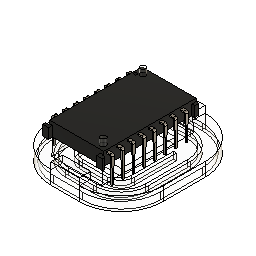
PMW3360 v12 (Autodesk Fusion 360 design; units mm, degrees)
Autodesk Fusion 360 part; units mm, degrees
sketch "Sketch1" plane through (0, 0, 0) normal (0, 0, 1) x (1, 0, 0) in component "Chip"
  line L0 (-4.55, 7.18) -> (4.55, 7.18)
  line L1 (4.55, 7.18) -> (4.55, -8.32)
  line L2 (4.55, -8.32) -> (-4.55, -8.32)
  line L3 (-4.55, -8.32) -> (-4.55, 7.18)
  line L4 (0, 7.18) -> (0, -8.32) construction
  dimension "d1" = 9.1
  dimension "d3" = 7.18
  dimension "d4" = 15.5
  constraint horizontal L0
  constraint vertical L1
  constraint horizontal L2
  constraint vertical L3
  constraint midpoint L0 L4.start
  constraint coincident L2 L4.end
  constraint vertical L4
  constraint coincident origin L4
  constraint coincident L4 origin
  measures "d1" distance of L0.start L0.end
  measures "d3" distance of L0 origin
  measures "d4" distance of L0.end L1.end
extrude "Extrude1" add sketch "Sketch1" against normal blind 0.5 makes body 1 in component "Chip"
sketch "Sketch2" plane through (0, 0, -0.5) normal (0, 0, -1) x (1, 0, 0) in component "Chip"
  line L0 (-4.55, 8.32) -> (4.55, 8.32)
  line L1 (4.55, 8.32) -> (4.55, -7.18)
  line L2 (4.55, -7.18) -> (-4.55, -7.18)
  line L3 (-4.55, -7.18) -> (-4.55, 8.32)
  line L4 (4.55, -7.18) -> (5.05, -7.18)
  line L5 (5.05, -7.18) -> (5.05, -6.48)
  line L6 (5.05, -6.48) -> (4.55, -6.48)
  line L7 (-4.55, -7.18) -> (-5.05, -7.18)
  line L8 (-5.05, -7.18) -> (-5.05, -6.68)
  line L9 (-4.85, -6.48) -> (-4.55, -6.48)
  line L10 (-4.55, -7.18) -> (-4.55, -6.48) construction
  line L11 (-5.05, -6.68) -> (-4.85, -6.48)
  line L12 (-4.55, 8.32) -> (-4.55, 8.52)
  line L13 (-4.55, 8.52) -> (-5.05, 8.52)
  line L14 (-5.05, 8.52) -> (-5.05, 9.02)
  line L15 (-5.05, 9.02) -> (-4.05, 9.02)
  line L16 (-4.05, 9.02) -> (-4.05, 8.32)
  line L17 (4.05, 8.32) -> (4.05, 9.02)
  line L18 (4.05, 9.02) -> (5.05, 9.02)
  line L19 (5.05, 9.02) -> (5.05, 8.72)
  line L20 (5.05, 8.72) -> (4.85, 8.52)
  line L21 (4.85, 8.52) -> (4.55, 8.52)
  line L22 (4.55, 8.52) -> (4.55, 8.32)
  dimension "d7" = 0.5
  dimension "d8" = 0.7
  dimension "d11" = 0.5
  dimension "d12" = 0.7
  dimension "d13" = 135
  dimension "d14" = 0.3
  dimension "d15" = 0.5
  dimension "d16" = 0.5
  dimension "d17" = 1
  dimension "d18" = 0.7
  dimension "d19" = 0.7
  dimension "d20" = 0.5
  dimension "d21" = 1
  dimension "d22" = 0.5
  dimension "d23" = 135
  dimension "d24" = 0.3
  constraint coincident L1.end L2.start
  constraint perpendicular L1 L4
  constraint perpendicular L4 L5
  constraint coincident L1 L6.end
  constraint perpendicular L1 L6
  constraint perpendicular L3 L7
  constraint perpendicular L7 L8
  constraint coincident L2.end L3.start
  constraint coincident L3 L9.end
  constraint perpendicular L3 L9
  constraint coincident L0.start L3.end
  constraint perpendicular L0 L12
  constraint perpendicular L3 L13
  constraint perpendicular L13 L14
  constraint perpendicular L14 L15
  constraint coincident L0 L16.end
  constraint perpendicular L0 L16
  constraint coincident L0 L17.start
  constraint perpendicular L0 L17
  constraint perpendicular L17 L18
  constraint perpendicular L18 L19
  constraint perpendicular L19 L21
  constraint coincident L0.end L1.start
  constraint vertical L22
  measures "d7" distance of L1.end L4.end
  measures "d8" distance of L4.end L5.end
  measures "d11" distance of L2.end L7.end
  measures "d12" distance of L2.end L9.end
  measures "d13" angle of L9 L11
  measures "d14" distance of L9.end L9.start
  measures "d15" distance of L12 L16
  measures "d16" distance of L13.end L14.end
  measures "d17" distance of L14.end L15.end
  measures "d18" distance of L15.end L16.end
  measures "d19" distance of L17.start L17.end
  measures "d20" distance of L18 L21
  measures "d21" distance of L17.end L18.end
  measures "d22" distance of L17 L22
  measures "d23" angle of L20 L21
  measures "d24" distance of L18.end L19.end
extrude "Extrude2" add sketch "Sketch2" along normal blind 1.71 bodies 1 in component "Chip"
ref_plane "WorkPlane1" through (0, 5.66, -1.105) normal (0, 1, 0) x (1, 0, 0) in component "Chip"
sketch "Sketch1 (2)" plane through (0, 5.66, -1.105) normal (0, 1, 0) x (1, 0, 0) in component "Lead"
  line L0 (-4.55, -1.105) -> (-4.55, -0.605) construction
  line L1 (-4.55, -0.605) -> (-5.15, -0.605)
  line L2 (-5.25, -0.505) -> (-5.25, 3.705)
  arc A0 (-5.25, -0.505) -> (-5.15, -0.605) centre (-5.15, -0.505) ccw
  line L3 (-4.55, -0.805) -> (-5.15, -0.805)
  arc A1 (-5.45, -0.505) -> (-5.15, -0.805) centre (-5.15, -0.505) ccw
  line L4 (-5.45, -0.505) -> (-5.45, 3.705)
  line L5 (-5.25, 3.705) -> (-5.45, 3.705)
  line L6 (-4.55, -0.805) -> (-4.55, -0.605)
  dimension "d28" = 0.7
  dimension "d29" = 0.1
  dimension "d30" = 4.31
  dimension "d31" = -0.2
  constraint coincident L0.end L1.start
  constraint perpendicular L0 L1
  constraint perpendicular L1 L2
  constraint tangent L1 A0
  constraint tangent L2 A0
  constraint perpendicular L1 L6
  measures "d28" distance of L0 L2
  measures "d29" radius of A0
  measures "d30" distance of L1 L2.end
extrude "Extrude1'" add sketch "Sketch1 (2)" along normal mid plane 0.5 separate body makes body 2 in component "Lead"
sketch "Sketch2 (2)" plane through (-5.45, 0, 0) normal (-1, 0, 0) x (0, -1, 0) in component "Lead"
  line L0 (8.32, 0) -> (-7.18, 0) construction
  line L1 (-5.41, -0.6) -> (-5.91, -0.6) construction
  line L2 (-5.91, -0.6) -> (-5.91, -4.81) construction
  line L3 (-5.91, -4.81) -> (-5.41, -4.81) construction
  line L4 (-5.41, -4.81) -> (-5.41, -0.6) construction
  line L5 (-5.91, -2) -> (-5.41, -2) construction
  line L6 (-5.91, -2) -> (-5.91, -4.81)
  line L7 (-5.91, -2) -> (-5.785, -2.216506)
  line L8 (-5.41, -2) -> (-5.535, -2.216506)
  line L9 (-5.535, -2.216506) -> (-5.535, -4.81)
  line L10 (-5.785, -4.81) -> (-5.785, -2.216506)
  line L11 (-5.41, -2) -> (-5.41, -4.81)
  line L12 (-5.535, -4.81) -> (-5.41, -4.81)
  line L13 (-5.91, -4.81) -> (-5.785, -4.81)
  dimension "d34" = 2
  dimension "d35" = 60
  dimension "d36" = 60
  dimension "d37" = 0.125
  dimension "d38" = 0.125
  constraint coincident L2 L5.start
  constraint coincident L4 L5.end
  constraint perpendicular L4 L5
  constraint perpendicular L5 L6
  constraint coincident L3 L9.end
  constraint perpendicular L3 L9
  constraint coincident L3 L10.start
  constraint vertical L10
  constraint coincident L2.end L3.start
  constraint coincident L3.end L4.start
  measures "d34" distance of L0 L5
  measures "d35" angle of L5 L7
  measures "d36" angle of L5 L8
  measures "d37" distance of L2 L10
  measures "d38" distance of L4 L9
extrude "Extrude2'" cut sketch "Sketch2 (2)" against normal up to surface (0.2 mm away) bodies 2 in component "Lead"
pattern_linear "愁3" [suppressed] in component "Chip"
mirror "MirrorComponent1" about plane through (0, 0, 0) normal (0, 0, 1) of bodies 2 makes body 3 in component "Lead(Mirror)"
hole "Hole1" at (-4.05, 5.66, 0) direction (0, 0, -1) diameter 0.5 depth 0.5 tip angle 180 bodies 1 in component "Chip"
sketch "Sketch1 (3)" plane through (0, 0, 0) normal (0, 0, 1) x (1, 0, 0) in component "Lens"
  line L0 (-2.375, 10.87) -> (2.375, 10.87)
  line L1 (9.425, 3.82) -> (9.425, -3.23)
  line L2 (2.375, -10.28) -> (-2.375, -10.28)
  line L3 (-9.425, -3.23) -> (-9.425, 3.82)
  line L4 (0, 10.87) -> (0, -10.28) construction
  arc A0 (-9.425, -3.23) -> (-2.375, -10.28) centre (-2.375, -3.23) ccw
  arc A1 (-2.375, 10.87) -> (-9.425, 3.82) centre (-2.375, 3.82) ccw
  arc A2 (9.425, 3.82) -> (2.375, 10.87) centre (2.375, 3.82) ccw
  arc A3 (2.375, -10.28) -> (9.425, -3.23) centre (2.375, -3.23) ccw
  point P0 (-9.425, 10.87)
  point P1 (9.425, 10.87)
  point P2 (9.425, -10.28)
  point P3 (0, 10.87)
  dimension "d50" = 18.85
  dimension "d51" = 21.15
  dimension "d52" = 10.87
  dimension "d53" = 7.05
  constraint horizontal L0
  constraint vertical L1
  constraint horizontal L2
  constraint vertical L3
  constraint coincident L2 L4.end
  constraint vertical L4
  constraint coincident L4 origin
  constraint tangent L2 A0
  constraint tangent L3 A0
  constraint coincident L0 P3
  constraint coincident P0 L3
  constraint coincident P0 L0
  constraint tangent L3 A1
  constraint tangent L0 A1
  constraint equal A0 A1
  constraint coincident P1 L0
  constraint coincident P1 L1
  constraint tangent L0 A2
  constraint tangent L1 A2
  constraint equal A0 A2
  constraint coincident P2 L1
  constraint coincident P2 L2
  constraint tangent L1 A3
  constraint tangent L2 A3
  constraint equal A0 A3
  constraint midpoint L0 P3
  constraint coincident P3 L4.start
  measures "d50" distance of P0 P1
  measures "d51" distance of P1 P2
  measures "d52" distance of L0 origin
  measures "d53" radius of A0
extrude "Extrude1''" add sketch "Sketch1 (3)" along normal blind 1.14 separate body makes body 4 in component "Lens"
sketch "Sketch2 (3)" plane through (0, 0, 0) normal (0, 0, -1) x (1, 0, 0) in component "Lens"
  line L0 (-9.425, -3.82) -> (-9.425, 3.23)
  arc A0 (-9.425, -3.82) -> (-2.375, -10.87) centre (-2.375, -3.82) ccw
  line L1 (2.375, -10.87) -> (-2.375, -10.87)
  arc A1 (2.375, -10.87) -> (9.425, -3.82) centre (2.375, -3.82) ccw
  line L2 (9.425, 3.23) -> (9.425, -3.82)
  arc A2 (9.425, 3.23) -> (2.375, 10.28) centre (2.375, 3.23) ccw
  line L3 (-2.375, 10.28) -> (2.375, 10.28)
  arc A3 (-2.375, 10.28) -> (-9.425, 3.23) centre (-2.375, 3.23) ccw
  arc A4 (-8.925, -3.82) -> (-2.375, -10.37) centre (-2.375, -3.82) ccw
  line L4 (2.375, -10.37) -> (-2.375, -10.37)
  arc A5 (2.375, -10.37) -> (8.925, -3.82) centre (2.375, -3.82) ccw
  line L5 (8.925, 3.23) -> (8.925, -3.82)
  arc A6 (8.925, 3.23) -> (2.375, 9.78) centre (2.375, 3.23) ccw
  line L6 (-2.375, 9.78) -> (2.375, 9.78)
  arc A7 (-2.375, 9.78) -> (-8.925, 3.23) centre (-2.375, 3.23) ccw
  line L7 (-8.925, -3.82) -> (-8.925, 3.23)
  line L8 (2.375, -8.47) -> (-2.375, -8.47)
  arc A8 (-7.025, -3.82) -> (-2.375, -8.47) centre (-2.375, -3.82) ccw
  line L9 (-7.025, -3.82) -> (-7.025, 3.23)
  arc A9 (-2.375, 7.88) -> (-7.025, 3.23) centre (-2.375, 3.23) ccw
  line L10 (-2.375, 7.88) -> (2.375, 7.88)
  arc A10 (7.025, 3.23) -> (2.375, 7.88) centre (2.375, 3.23) ccw
  line L11 (7.025, 3.23) -> (7.025, -3.82)
  arc A11 (2.375, -8.47) -> (7.025, -3.82) centre (2.375, -3.82) ccw
  line L12 (2.375, -7.97) -> (-2.375, -7.97)
  arc A12 (-6.525, -3.82) -> (-2.375, -7.97) centre (-2.375, -3.82) ccw
  line L13 (-6.525, -3.82) -> (-6.525, 3.23)
  arc A13 (-2.375, 7.38) -> (-6.525, 3.23) centre (-2.375, 3.23) ccw
  line L14 (-2.375, 7.38) -> (2.375, 7.38)
  arc A14 (6.525, 3.23) -> (2.375, 7.38) centre (2.375, 3.23) ccw
  line L15 (6.525, 3.23) -> (6.525, -3.82)
  arc A15 (2.375, -7.97) -> (6.525, -3.82) centre (2.375, -3.82) ccw
  line L16 (-4.625, -3.82) -> (-4.625, 3.23)
  arc A16 (-2.375, 5.48) -> (-4.625, 3.23) centre (-2.375, 3.23) ccw
  line L17 (-2.375, 5.48) -> (2.375, 5.48)
  arc A17 (4.625, 3.23) -> (2.375, 5.48) centre (2.375, 3.23) ccw
  line L18 (4.625, 3.23) -> (4.625, -3.82)
  line L19 (-4.125, -3.82) -> (-4.125, 3.23)
  arc A18 (-2.375, 4.98) -> (-4.125, 3.23) centre (-2.375, 3.23) ccw
  line L20 (-2.375, 4.98) -> (2.375, 4.98)
  arc A19 (4.125, 3.23) -> (2.375, 4.98) centre (2.375, 3.23) ccw
  line L21 (4.125, 3.23) -> (4.125, -3.82)
  line L22 (-4.625, -3.82) -> (-4.125, -3.82)
  line L23 (4.125, -3.82) -> (4.625, -3.82)
  line L24 (-9.425, -3.82) -> (9.425, -3.82) construction
  line L25 (-2.225, -6.07) -> (2.225, -6.07)
  line L26 (2.225, -6.07) -> (2.225, 3.08)
  line L27 (2.225, 3.08) -> (-2.225, 3.08)
  line L28 (-2.225, 3.08) -> (-2.225, -6.07)
  line L29 (0, -6.07) -> (0, 3.08) construction
  dimension "d56" = 0.5
  dimension "d57" = -2.4
  dimension "d58" = -2.9
  dimension "d61" = 0.5
  dimension "d63" = 1.9
  dimension "d64" = 1.9
  dimension "d65" = 1.9
  dimension "d66" = 1.9
  constraint parallel L0 L16
  constraint concentric A3 A16
  constraint parallel L3 L17
  constraint concentric A2 A17
  constraint parallel L2 L18
  constraint tangent A17 L18
  constraint tangent L16 A16
  constraint tangent A16 L17
  constraint tangent L17 A17
  constraint parallel L0 L19
  constraint concentric A3 A18
  constraint parallel L3 L20
  constraint concentric A2 A19
  constraint parallel L2 L21
  constraint tangent L19 A18
  constraint tangent A18 L20
  constraint tangent L20 A19
  constraint tangent A19 L21
  constraint perpendicular L19 L22
  constraint perpendicular L21 L23
  constraint coincident L0.start A0.start
  constraint coincident A1.end L2.end
  constraint coincident L16.start L24
  constraint coincident L21.end L24
  constraint horizontal L25
  constraint vertical L26
  constraint horizontal L27
  constraint vertical L28
  constraint midpoint L25 L29.start
  constraint coincident L27 L29.end
  constraint vertical L29
  constraint coincident origin L29
  measures "d61" distance of L16 L19
  measures "d63" distance of L19 L28
  measures "d64" distance of L20 L27
  measures "d65" distance of L13 L16
  measures "d66" distance of L12 L25
extrude "Extrude2''" add sketch "Sketch2 (3)" along normal blind 1.14 bodies 4 in component "Lens"
sketch "Sketch3" plane through (0, -10.28, 0) normal (0, -1, 0) x (1, 0, 0) in component "Lens"
  line L0 (2.375, -1.14) -> (2.375, 1.14) construction
  line L1 (2.375, 1.14) -> (-2.375, 1.14)
  line L2 (-2.375, 1.14) -> (-2.375, -1.14) construction
  line L3 (-2.375, -1.14) -> (2.375, -1.14) construction
  line L4 (-2.375, 1.14) -> (-2.375, 2.28)
  line L5 (-2.375, 2.28) -> (2.375, 2.28)
  line L6 (2.375, 2.28) -> (2.375, 1.14)
  dimension "d69" = 1.14
  constraint coincident L1.end L2.start
  constraint perpendicular L1 L4
  constraint perpendicular L4 L5
  constraint coincident L0.end L1.start
  constraint vertical L6
  measures "d69" distance of L1.end L4.end
extrude "Extrude3" add sketch "Sketch3" against normal up to surface (21.15 mm away) bodies 4 in component "Lens"
sketch "Sketch4" plane through (0, -10.28, 0) normal (0, -1, 0) x (1, 0, 0) in component "Lens"
  line L0 (2.375, -1.14) -> (2.375, 1.14) construction
  line L1 (2.375, 1.14) -> (2.375, 2.28)
  line L2 (2.375, 2.28) -> (-2.375, 2.28)
  line L3 (-2.375, 2.28) -> (-2.375, 1.14)
  line L4 (-2.375, 1.14) -> (-2.375, -1.14) construction
  line L5 (-2.375, -1.14) -> (2.375, -1.14) construction
  line L6 (9.425, -1.14) -> (9.425, 1.14) construction
  line L7 (9.425, 1.14) -> (2.375, 1.14)
  line L8 (2.375, 1.14) -> (2.375, -1.14) construction
  line L9 (2.375, -1.14) -> (9.425, -1.14) construction
  line L10 (-2.375, -1.14) -> (-2.375, 1.14) construction
  line L11 (-2.375, 1.14) -> (-9.425, 1.14)
  line L12 (-9.425, 1.14) -> (-9.425, -1.14) construction
  line L13 (-9.425, -1.14) -> (-2.375, -1.14) construction
  line L14 (-4.235, 1.14) -> (-4.235, 1.71)
  line L15 (-4.235, 1.71) -> (-4.235, 5.57)
  line L16 (-4.235, 5.57) -> (-2.375, 5.57)
  line L17 (-2.375, 5.57) -> (-2.375, 3.925)
  line L18 (-2.375, 3.925) -> (2.375, 3.925)
  line L19 (2.375, 3.925) -> (2.375, 5.57)
  line L20 (2.375, 5.57) -> (4.235, 5.57)
  line L21 (4.235, 5.57) -> (4.235, 1.14)
  line L22 (-2.375, 3.925) -> (-2.375, 2.28) construction
  dimension "d72" = 8.47
  dimension "d73" = 6.71
  constraint coincident L11 L14.start
  constraint perpendicular L11 L14
  constraint perpendicular L11 L15
  constraint perpendicular L15 L16
  constraint perpendicular L16 L17
  constraint perpendicular L17 L18
  constraint coincident L7 L21.end
  constraint perpendicular L7 L21
  constraint horizontal L20
  constraint collinear L3 L17
  constraint collinear L1 L19
  constraint collinear L16 L20
  constraint equal L16 L20
  constraint coincident L18.end L19.start
  constraint coincident L2.end L3.start
  constraint perpendicular L2 L22
  constraint equal L17 L22
  measures "d72" distance of L15 L21
  measures "d73" distance of L9 L20
extrude "Extrude4" add sketch "Sketch4" against normal up to surface (21.15 mm away) bodies 4 in component "Lens"
extrude "Extrude5" cut sketch "Sketch4" against normal up to surface (1.96 mm away) bodies 4 in component "Lens"
extrude "Extrude6" cut sketch "Sketch4" against normal up to surface (3.69 mm away) from surface at -17.46 bodies 4 in component "Lens"
sketch "Sketch5" plane through (0, 0, 5.57) normal (0, 0, 1) x (-1, 0, 0) in component "Lens"
  circle A0 centre (3.35, -6.18) radius 0.45
  ellipse E0 centre (-3.48, 7.36) end of major axis (-3.126447, 7.713553) minor radius 0.375
  line L0 (-3.833553, 7.006447) -> (-3.126447, 7.713553)
  line L1 (-3.214835, 7.094835) -> (-3.745165, 7.625165)
  line L2 (-4.235, 8.32) -> (-4.235, -7.18)
  dimension "d81" = 0.9
  dimension "d82" = 6.18
  dimension "d83" = 3.35
  dimension "d87" = 45
  dimension "d88" = 0.75
  dimension "d89" = 1
  dimension "d90" = 13.54
  dimension "d91" = 6.83
  measures "d81" diameter of A0
  measures "d82" vertical distance of origin A0.centre
  measures "d83" horizontal distance of origin A0.centre
  measures "d87" angle of L0 L2
  measures "d89" distance of E0
  measures "d90" distance of A0.centre E0.centre
  measures "d91" distance of A0.centre E0.centre
extrude "Extrude7" add sketch "Sketch5" along normal blind 1.75 bodies 4 in component "Lens"
sketch "Sketch6" plane through (0, -8.32, 0) normal (0, -1, 0) x (1, 0, 0) in component "Lens"
  line L0 (2.375, 5.57) -> (2.375, 3.925) construction
  line L1 (2.375, 3.925) -> (-2.375, 3.925)
  line L2 (-2.375, 3.925) -> (-2.375, 5.57) construction
  line L3 (-2.375, 5.57) -> (-4.235, 5.57) construction
  line L4 (-4.235, 5.57) -> (-4.235, 1.14) construction
  line L5 (-4.235, 1.14) -> (-2.375, 1.14) construction
  line L6 (-2.375, 1.14) -> (-2.375, 2.28) construction
  line L7 (-2.375, 2.28) -> (2.375, 2.28) construction
  line L8 (2.375, 2.28) -> (2.375, 1.14) construction
  line L9 (2.375, 1.14) -> (4.235, 1.14) construction
  line L10 (4.235, 1.14) -> (4.235, 5.57) construction
  line L11 (4.235, 5.57) -> (2.375, 5.57) construction
  line L12 (-2.9, 7.32) -> (-3.8, 7.32)
  line L13 (-3.8, 5.57) -> (-2.9, 5.57) construction
  line L14 (3.921942, 7.32) -> (3.038058, 7.32)
  line L15 (3.038058, 5.57) -> (3.921942, 5.57) construction
  line L16 (-4.235, 1.14) -> (-4.002834, 5.57)
  line L17 (4.235, 1.14) -> (4.002834, 5.57)
  line L18 (-4.002834, 5.57) -> (-3.8, 5.57)
  line L19 (-3.8, 7.32) -> (-3.8, 5.57)
  line L20 (-2.9, 7.32) -> (-2.9, 5.57)
  line L21 (4.002834, 5.57) -> (3.921942, 5.57)
  line L22 (3.921942, 7.32) -> (3.921942, 5.57)
  line L23 (3.038058, 7.32) -> (3.038058, 5.57)
  line L24 (-2.461211, 5.57) -> (-2.375, 3.925)
  line L25 (2.375, 3.925) -> (2.461211, 5.57)
  line L26 (-4.235, 1.14) -> (-4.235, 7.32)
  line L27 (-4.235, 7.32) -> (-3.8, 7.32)
  line L28 (-2.9, 7.32) -> (3.038058, 7.32)
  line L29 (3.921942, 7.32) -> (4.235, 7.32)
  line L30 (4.235, 7.32) -> (4.235, 1.14)
  line L31 (-2.9, 5.57) -> (-2.461211, 5.57)
  line L32 (2.461211, 5.57) -> (3.038058, 5.57)
  dimension "d94" = 87
  dimension "d95" = 87
  dimension "d96" = 87
  dimension "d97" = 87
  constraint coincident L4.end L5.start
  constraint coincident L9.end L10.start
  constraint coincident L13.start L18.end
  constraint coincident L12.end L19.start
  constraint coincident L12.start L20.start
  constraint coincident L13.end L20.end
  constraint coincident L1.end L2.start
  constraint coincident L0.end L1.start
  constraint perpendicular L5 L26
  constraint perpendicular L22 L29
  constraint vertical L30
  constraint horizontal L27
  measures "d94" angle of L9 L17
  measures "d95" angle of L5 L16
  measures "d96" angle of L1 L24
  measures "d97" angle of L1 L25
extrude "Extrude8" cut sketch "Sketch6" against normal up to surface (15.5 mm away) bodies 4 in component "Lens"
sketch "Sketch10" plane through (-9.425, 0, 0) normal (-1, 0, 0) x (0, -1, 0) in component "Lens"
  line L0 (-7.18, 5.57) -> (-7.18, 1.14) construction
  line L1 (-7.18, 1.14) -> (8.32, 1.14) construction
  line L2 (8.32, 1.14) -> (8.32, 5.57) construction
  line L3 (8.32, 5.57) -> (-7.18, 5.57) construction
  line L4 (-5.73, 7.32) -> (-6.63, 7.32) construction
  line L5 (-6.63, 5.57) -> (-5.73, 5.57) construction
  line L6 (7.801942, 7.32) -> (6.918058, 7.32) construction
  line L7 (6.918058, 5.57) -> (7.801942, 5.57) construction
  line L8 (-7.18, 1.14) -> (-6.792425, 5.57)
  line L9 (7.932425, 5.57) -> (8.32, 1.14)
  line L10 (-4.392425, 5.57) -> (-4.00485, 1.14)
  line L11 (6.732425, 5.57) -> (6.34485, 1.14)
  line L12 (-7.18, 1.14) -> (-7.18, 7.82)
  line L13 (-7.18, 7.82) -> (8.32, 7.82)
  line L14 (8.32, 7.82) -> (8.32, 1.14)
  line L15 (-4.00485, 1.14) -> (6.34485, 1.14)
  line L16 (-6.792425, 5.57) -> (-6.63, 5.57)
  line L17 (-6.63, 5.57) -> (-6.63, 7.32)
  line L18 (-6.63, 7.32) -> (-5.73, 7.32)
  line L19 (-5.73, 7.32) -> (-5.73, 5.57)
  line L20 (-5.73, 5.57) -> (-4.392425, 5.57)
  line L21 (6.732425, 5.57) -> (6.918058, 5.57)
  line L22 (6.918058, 7.32) -> (6.918058, 5.57)
  line L23 (6.918058, 7.32) -> (7.801942, 7.32)
  line L24 (7.801942, 7.32) -> (7.801942, 5.57)
  line L25 (7.932425, 5.57) -> (7.801942, 5.57)
  line L26 (8.32, 3.925) -> (-7.18, 3.925)
  dimension "d100" = 85
  dimension "d101" = 85
  dimension "d102" = 85
  dimension "d103" = 85
  dimension "d104" = 2.4
  dimension "d105" = 1.2
  dimension "d106" = 0.5
  constraint coincident L0.end L1.start
  constraint coincident L1.end L2.start
  constraint perpendicular L1 L12
  constraint perpendicular L12 L13
  constraint vertical L14
  constraint coincident L5.start L16.end
  constraint coincident L4.end L17.end
  constraint coincident L4.start L18.end
  constraint coincident L5.end L19.end
  measures "d100" angle of L1 L8
  measures "d101" angle of L1 L9
  measures "d102" angle of L1 L10
  measures "d103" angle of L1 L11
  measures "d106" distance of L4 L13
extrude "Extrude9" cut sketch "Sketch10" along normal up to surface contours L8 L12 L26 | L8 L9 L10 L11 L12 L13 L14 L16 L17 L18 L19 L20 L21 L22 L23 L24 L25 L26 | L9 L14 L26 picked at (-7.098781, 2.996667) picked at (-1.068122, 6.736667) picked at (8.238781, 2.996667) end surface through (4.235, -8.32, 1.14) normal (0.99862953, 0, 0.05233596) offset 0 bodies 4 in component "Lens"
combine "Combine1" operation cut target body 1 tool bodies 4 body 4 seen with x (1, 0, 0) y (0, 1, 0) z (0, 0, 1) at (0, 0, -6.27) keep tools in component "Chip"
hole "Hole2" at (3.48, -7.36, 0) direction (0, 0, -1) diameter 1 depth 2.21 tip angle 180 bodies 1 in component "Chip"
component "Chip" placed x (1, 0, 0) y (0, 1, 0) z (0, 0, 1) at (0, 0, 0)
component "Lens" placed x (1, 0, 0) y (0, 1, 0) z (0, 0, 1) at (0, 0, -6.27)
component "Lead" placed x (1, 0, 0) y (0, 1, 0) z (0, 0, 1) at (0, 0, 0) in component "Chip"
component "Lead" placed x (1, 0, 0) y (0, 1, 0) z (0, 0, 1) at (0, -1.78, 0) in component "Chip"
component "Lead" placed x (1, 0, 0) y (0, 1, 0) z (0, 0, 1) at (0, -3.56, 0) in component "Chip"
component "Lead" placed x (1, 0, 0) y (0, 1, 0) z (0, 0, 1) at (0, -5.34, 0) in component "Chip"
component "Lead" placed x (1, 0, 0) y (0, 1, 0) z (0, 0, 1) at (0, -7.12, 0) in component "Chip"
component "Lead" placed x (1, 0, 0) y (0, 1, 0) z (0, 0, 1) at (0, -8.9, 0) in component "Chip"
component "Lead" placed x (1, 0, 0) y (0, 1, 0) z (0, 0, 1) at (0, -10.68, 0) in component "Chip"
component "Lead" placed x (1, 0, 0) y (0, 1, 0) z (0, 0, 1) at (0, -12.46, 0) in component "Chip"
component "Lead(Mirror)" placed x (-1, 0, 0) y (0, 1, 0) z (0, 0, -1) at (0, -0.89, 0) in component "Chip"
component "Lead(Mirror)" placed x (-1, 0, 0) y (0, 1, 0) z (0, 0, -1) at (0, -2.67, 0) in component "Chip"
component "Lead(Mirror)" placed x (-1, 0, 0) y (0, 1, 0) z (0, 0, -1) at (0, -4.45, 0) in component "Chip"
component "Lead(Mirror)" placed x (-1, 0, 0) y (0, 1, 0) z (0, 0, -1) at (0, -6.23, 0) in component "Chip"
component "Lead(Mirror)" placed x (-1, 0, 0) y (0, 1, 0) z (0, 0, -1) at (0, -8.01, 0) in component "Chip"
component "Lead(Mirror)" placed x (-1, 0, 0) y (0, 1, 0) z (0, 0, -1) at (0, -9.79, 0) in component "Chip"
component "Lead(Mirror)" placed x (-1, 0, 0) y (0, 1, 0) z (0, 0, -1) at (0, -11.57, 0) in component "Chip"
component "Lead(Mirror)" placed x (-1, 0, 0) y (0, 1, 0) z (0, 0, -1) at (0, -13.35, 0) in component "Chip"
equation "d4 = 16.2 mm - 0.7 mm"
